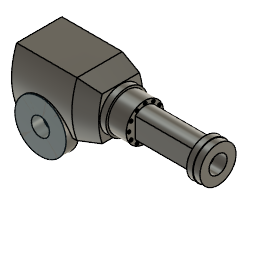
mechanical_joint (Autodesk Fusion 360 design; units mm, degrees)
part number: 2026-05-06-17-57-45-139
Autodesk Fusion 360 part; units mm, degrees
sketch "Sketch1" plane through (0, 0, 0) normal (1, 0, 0) x (0, 1, 0)
  line L0 (0, 0) -> (0, 45)
  line L1 (0, 0) -> (0, -45)
  line L2 (0, 45) -> (37.5, 45)
  line L3 (0, 45) -> (-37.5, 45)
  line L4 (0, -45) -> (37.5, -45)
  line L5 (0, -45) -> (-37.5, -45)
  arc A0 (37.5, -45) -> (37.5, 45) centre (-79.119, 0) ccw
  arc A1 (-37.5, 45) -> (-37.5, -45) centre (79.119, 0) ccw
  dimension "d1" = 45
  dimension "d2" = 45
  dimension "d3" = 37.5
  dimension "d4" = 37.5
  dimension "d6" = 125
  constraint coincident L0.start L1.start
  constraint vertical L0
  constraint parallel L0 L1
  constraint perpendicular L0 L2
  constraint perpendicular L0 L3
  constraint perpendicular L1 L4
  constraint perpendicular L1 L5
  constraint symmetric L0 L2.end L3.end
  constraint symmetric L0 L4.end L5.end
  constraint symmetric L0 A0 A1
  measures "d1" distance of L0.start L0.end
  measures "d2" distance of L0.start L1.end
  measures "d3" distance of L0.end L2.end
  measures "d4" distance of L0.end L3.end
  measures "d6" radius of A0
extrude "Extrude1" add sketch "Sketch1" along normal blind 100
sketch "Sketch2" plane through (0, 0, 0) normal (1, 0, 0) x (0, 1, 0)
extrude "Extrude2" add 1 faces at (100, -15.1807, -3.0661) along direction (1, 0, 0) blind 35 draft -15
sketch "Sketch3" plane through (0, 0, 0) normal (-1, 0, 0) x (0, -1, 0)
  line L0 (37.5, 45) -> (-37.5, 45)
  arc A0 (-37.5, 45) -> (-37.5, -45) centre (79.119, 0) ccw
  line L1 (-37.5, -45) -> (37.5, -45)
  arc A1 (37.5, -45) -> (37.5, 45) centre (-79.119, 0) ccw
sketch "Sketch4" plane through (135, 0, 0) normal (1, 0, 0) x (0, 1, 0)
  line L0 (30.8786, 35.6218) -> (-30.8786, 35.6218)
  arc A0 (-30.8786, 35.6218) -> (-30.8786, -35.6218) centre (79.119, 0) ccw
  line L1 (-30.8786, -35.6218) -> (30.8786, -35.6218)
  arc A1 (30.8786, -35.6218) -> (30.8786, 35.6218) centre (-79.119, 0) ccw
  circle A2 centre (0, 0) radius 34.5
  dimension "d11" = 69
  constraint coincident A2.centre origin
  measures "d11" diameter of A2
extrude "Extrude3" add sketch "Sketch4" along normal blind 10 contours A2
sketch "Sketch5" plane through (145, 0, 0) normal (1, 0, 0) x (0, 1, 0)
  circle A0 centre (0, 0) radius 34.5
  circle A1 centre (0, 0) radius 31
  dimension "d14" = 62
  constraint coincident A0.centre A1.centre
  measures "d14" diameter of A1
extrude "Extrude4" add sketch "Sketch5" along normal blind 30 contours A1
sketch "Sketch6" plane through (175, 0, 0) normal (1, 0, 0) x (0, 1, 0)
  circle A0 centre (0, 0) radius 31
  line L0 (0, 0) -> (27, 0)
  circle A1 centre (27, 0) radius 2.5
  circle A2 centre (27, 0) radius 1.5
  dimension "d17" = 27
  dimension "d18" = 5
  dimension "d19" = -1
  constraint coincident A0.centre L0.start
  constraint horizontal L0
  constraint coincident L0.end A1.centre
  measures "d17" distance of A0.centre L0.end
  measures "d18" diameter of A1
extrude "Extrude5" add sketch "Sketch6" along normal blind 1 contours A1
sketch "Sketch7" plane through (175, 0, 0) normal (1, 0, 0) x (0, 1, 0)
  circle A0 centre (0, 0) radius 31
  circle A1 centre (27, 0) radius 2.5
sketch "Sketch8" plane through (175, 0, 0) normal (1, 0, 0) x (0, 1, 0)
sketch "Sketch9" plane through (175, 0, 0) normal (1, 0, 0) x (0, 1, 0)
pattern_circular "C-Pattern1" count 12 over 360 about axis through (1.75, 0, 0) along (1, 0, 0) of "Extrude5"
sketch "Sketch10" plane through (175, 0, 0) normal (1, 0, 0) x (0, 1, 0)
  line L0 (0, 0) -> (16, 0)
  line L1 (16, 0) -> (16, 17)
  line L2 (16, 0) -> (16, -17)
  line L3 (0, 0) -> (0, -10)
  line L4 (-16, 0) -> (-16, 17)
  line L5 (-16, 0) -> (-16, -17)
  arc A0 (16, 17) -> (-16, 17) centre (0, 1.9003) ccw
  arc A1 (-16, -17) -> (16, -17) centre (0, -1.9003) ccw
  dimension "d24" = 16
  dimension "d25" = 17
  dimension "d26" = 17
  dimension "d27" = 22
  dimension "d28" = 22
  constraint coincident L0.start L3.start
  constraint horizontal L0
  constraint perpendicular L0 L1
  constraint perpendicular L0 L2
  constraint perpendicular L0 L3
  constraint symmetric L0.end L3 L4.start
  constraint symmetric L1.end L3 L4.end
  constraint symmetric L2.end L3 L5.end
  measures "d24" distance of L0.start L0.end
  measures "d25" distance of L0.end L1.end
  measures "d26" distance of L0.end L2.end
  measures "d27" radius of A0
  measures "d28" radius of A1
extrude "Extrude6" add sketch "Sketch10" along normal blind 100
sketch "Sketch11" plane through (275, 0, 0) normal (1, 0, 0) x (0, 1, 0)
  line L0 (-16, 17) -> (-16, -17)
  arc A0 (-16, -17) -> (16, -17) centre (0, -1.9003) ccw
  line L1 (16, -17) -> (16, 17)
  arc A1 (16, 17) -> (-16, 17) centre (0, 1.9003) ccw
  circle A2 centre (0, 0) radius 30.9877
  constraint coincident A2.centre origin
extrude "Extrude7" add sketch "Sketch11" along normal blind 10 contours L0 A0 L1 A1 | A2
sketch "Sketch12" plane through (285, 0, 0) normal (1, 0, 0) x (0, 1, 0)
  circle A0 centre (0, 0) radius 30.9877
  circle A1 centre (0, 0) radius 29.9877
  dimension "d33" = -1
extrude "Extrude8" add sketch "Sketch12" along normal blind 1 contours A1
extrude "Extrude9" add 1 faces at (286, 6.5805, -3.169) along direction (1, 0, 0) blind 10
sketch "Sketch13" plane through (0, 0, 0) normal (0, 1, 0) x (1, 0, 0)
ref_plane "WorkPlane1" through (0, -37.5, 45) normal (0, -1, 0) x (1, 0, 0)
sketch "Sketch14" plane through (0, -37.5, 0) normal (0, -1, 0) x (-1, 0, 0)
  circle A0 centre (-50, 45) radius 42.5
  dimension "d38" = 85
  measures "d38" diameter of A0
extrude "Extrude10" add sketch "Sketch14" along normal mid plane 21
sketch "Sketch15" plane through (0, -27, 0) normal (0, 1, 0) x (-1, 0, 0)
  line L0 (-7.5, -45) -> (-92.5, -45)
  arc A0 (-92.5, -45) -> (-7.5, -45) centre (-50, -45) ccw
  line L1 (-50, -45) -> (-50, -75)
  line L2 (-70, -45) -> (-70, -75)
  line L3 (-30, -45) -> (-30, -75)
  arc A1 (-70, -75) -> (-30, -75) centre (-50, -60) ccw
  line L4 (-70, -45) -> (-50, -45)
  line L5 (-50, -45) -> (-30, -45)
  line L6 (-70, -75) -> (-50, -75)
  line L7 (-30, -75) -> (-50, -75)
  dimension "d41" = 30
  dimension "d42" = 20
  dimension "d43" = -20
  dimension "d44" = 25
  constraint coincident A0.centre L1.start
  constraint perpendicular L0 L1
  constraint perpendicular L1 L4
  constraint perpendicular L3 L5
  constraint perpendicular L1 L6
  constraint perpendicular L1 L7
  measures "d41" distance of A0.centre L1.end
  measures "d44" radius of A1
extrude "Extrude11" add sketch "Sketch15" along normal blind 35 contours L0 L1 L3 L5 L7 | L0 L1 L2 L4 L6 | A1 L6 L7
sketch "Sketch16" plane through (70, 0, 0) normal (1, 0, 0) x (0, 1, 0)
  line L0 (-27, -45) -> (-27, -75)
  line L1 (-27, -75) -> (8, -75)
  line L2 (8, -75) -> (8, -45)
  line L3 (8, -45) -> (-27, -45)
  line L4 (8, -45) -> (33, -45)
  line L5 (8, -45) -> (8, -87)
  arc A0 (8, -87) -> (33, -45) centre (-21.8393, -40.7981) ccw
  dimension "d47" = 25
  dimension "d48" = 42
  dimension "d49" = 55
  constraint coincident L2.end L3.start
  constraint perpendicular L2 L4
  constraint perpendicular L1 L5
  measures "d47" distance of L2.end L4.end
  measures "d48" distance of L2.end L5.end
  measures "d49" radius of A0
extrude "Extrude12" add sketch "Sketch16" against normal blind 40 contours L2 L4 L5 A0
sketch "Sketch17" plane through (0, 8, 0) normal (0, -1, 0) x (1, 0, 0)
  arc A0 (30, -75) -> (70, -75) centre (50, -60) ccw
  line L0 (30, -75) -> (30, -87)
  line L1 (30, -87) -> (70, -87)
  line L2 (70, -87) -> (70, -75)
extrude "Extrude13" cut sketch "Sketch17" against normal blind 40
sketch "Sketch18" plane through (296, 0, 0) normal (1, 0, 0) x (0, 1, 0)
  circle A0 centre (0, 0) radius 29.9877
  circle A1 centre (0, 0) radius 15
  dimension "d54" = 30
  constraint coincident A0.centre A1.centre
  measures "d54" diameter of A1
extrude "Extrude14" cut sketch "Sketch18" against normal blind 20 contours A1
sketch "Sketch19" plane through (0, -48, 0) normal (0, -1, 0) x (1, 0, 0)
  circle A0 centre (50, -45) radius 42.5
  circle A1 centre (50, -45) radius 15
  dimension "d57" = 30
  constraint concentric A0 A1
  measures "d57" diameter of A1
extrude "Extrude15" cut sketch "Sketch19" against normal blind 19 contours A1
sketch "Sketch20" plane through (0, -48, 0) normal (0, -1, 0) x (1, 0, 0)
  circle A0 centre (50, -45) radius 15
  circle A1 centre (50, -45) radius 42.5
equation "d39 = ( 21 / 2 ) * 1 mm"
